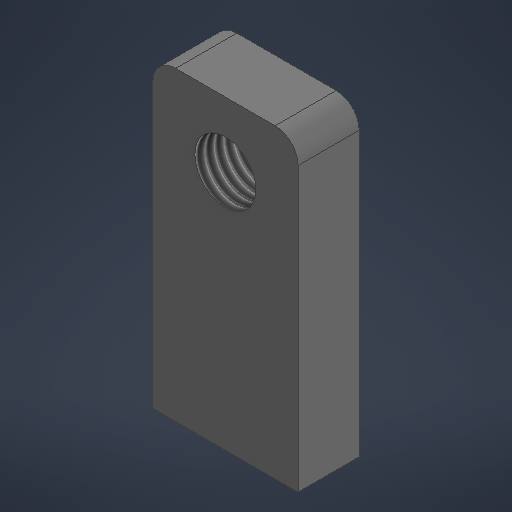
# Autodesk Inventor part: Kengyel2
Saved by Autodesk Inventor 2025 (Build 290162010, 162A)
## iProperties
Created: 2025-02-13
Part Number: Kengyel2
Material: Generic
Document SubType Name: Modeling
Designer: petruska.milan
Density: 1 g/cm^3
Appearance: Default
Author: petruska.milan
Autodesk Inventor part; units mm, degrees
ref_plane "YZ Plane" through (0, 0, 0) normal (1, 0, 0) x (0, 1, 0)
ref_plane "XZ Plane" through (0, 0, 0) normal (0, 1, 0) x (-1, 0, 0)
ref_plane "XY Plane" through (0, 0, 0) normal (0, 0, 1) x (1, 0, 0)
sketch "Sketch2" plane through (0, 0, 0) normal (0, 0, 1) x (1, 0, 0)
  line L0 (-9.5, -20) -> (9.5, -20)
  line L1 (9.5, -20) -> (9.5, 17)
  line L2 (6.5, 20) -> (-6.5, 20)
  line L3 (-9.5, 17) -> (-9.5, -20)
  line L4 (-9.5, -20) -> (9.5, 20) construction
  line L5 (9.5, -20) -> (-9.5, 20) construction
  arc A0 (-6.5, 20) -> (-9.5, 17) centre (-6.5, 17) ccw
  arc A1 (9.5, 17) -> (6.5, 20) centre (6.5, 17) ccw
  line L6 (0, 20) -> (0, 11.5)
  circle A2 centre (0, 11.5) radius 4
  point P0 (0, 0)
  dimension "d7" = 19
  dimension "d8" = 40
  dimension "d9" = 3
  dimension "d10" = 8.5
  dimension "d11" = 8
  constraints: 14 end point, 4 point on circle, 4 point on line, 4 tangent, 3 centre point, 3 midpoint, 2 parallel, 1 coincident, 1 equal radius, 1 horizontal, 1 perpendicular, 1 vertical
  measures "d7" distance of L5.end L4.end
  measures "d8" distance of L4.end L0.end
  measures "d9" radius of A0
  measures "d10" distance of L6.start L6.end
  measures "d11" diameter of A2
extrude "Extrusion2" add sketch "Sketch2" along normal blind 8
thread "Thread1" size "M8x1.25" class "6H" standard "ANSI Metric M Profile" full length
body "Solid2"
